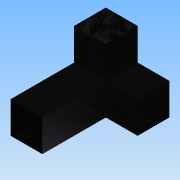
# Autodesk Inventor part: BlackPuzzlePiece
Saved by Autodesk Inventor 2015 (Build 190159000, 159)
## iProperties
Created: 2016-10-14
Part Number: BlackPuzzlePiece
Material: Generic
Document SubType Name: Modeling
Designer: Aniket Pant
Density: 1 g/cm^3
Appearance: Default
Author: Aniket Pant
Autodesk Inventor part; units mm, degrees
ref_plane "YZ Plane" through (0, 0, 0) normal (1, 0, 0) x (0, 1, 0)
ref_plane "XZ Plane" through (0, 0, 0) normal (0, 1, 0) x (-1, 0, 0)
ref_plane "XY Plane" through (0, 0, 0) normal (0, 0, 1) x (1, 0, 0)
sketch "Sketch1" plane through (0, 0, 0) normal (0, 1, 0) x (-1, 0, 0)
  line L0 (0, 0) -> (0, -76.2)
  line L1 (0, -76.2) -> (-50.8, -76.2)
  line L2 (-25.4, 0) -> (0, 0)
  line L3 (0, 0) -> (-25.4, 0)
  line L4 (-25.4, 0) -> (-25.4, -50.8)
  line L5 (-25.4, -50.8) -> (-50.8, -50.8)
  line L6 (-50.8, -50.8) -> (-50.8, -76.2)
  dimension "d0" = 76.2
  dimension "d1" = 50.8
  dimension "d11" = 25.4
  dimension "d12" = 50.8
  dimension "d13" = 25.4
  constraints: 14 end point, 4 perpendicular, 1 collinear, 1 vertical
  measures "d0" distance of L0.start L0.end
  measures "d1" distance of L0.end L1.end
  measures "d11" distance of L0.start L2.start
  measures "d12" distance of L2.start L4.end
  measures "d13" distance of L4.end L5.end
extrude "Extrusion1" add sketch "Sketch1" along normal blind 25.4
sketch "Sketch2" plane through (0, 25.4, 0) normal (0, 1, 0) x (1, 0, 0)
  line L0 (0, 76.2) -> (25.4, 76.2)
  line L1 (50.8, 76.2) -> (0, 76.2) projected
  line L2 (25.4, 76.2) -> (25.4, 50.8)
  line L3 (25.4, 50.8) -> (0, 50.8)
  line L4 (0, 76.2) -> (0, 0) projected
  line L5 (0, 50.8) -> (0, 76.2)
  dimension "d6" = 25.4
  dimension "d7" = 25.4
  dimension "d8" = 25.4
  constraints: 8 end point, 1 collinear, 1 midpoint, 1 perpendicular, 1 point on line
  measures "d6" distance of L0.start L0.end
  measures "d7" distance of L0.end L2.end
  measures "d8" distance of L2.end L3.end
extrude "Extrusion2" add sketch "Sketch2" along normal blind 25.4
body "Solid1"
